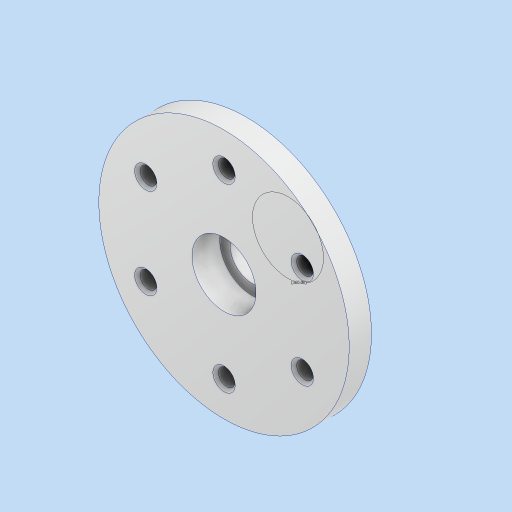
# Autodesk Inventor part: output pin holder
Saved by Autodesk Inventor 2023 (Build 270158000, 158)
## iProperties
Created: 2023-01-17
Part Number: output pin holder
Material: Aluminum 6061
Document SubType Name: Modeling
Designer: caden
Density: 2.7 g/cm^3
Appearance: Aluminum - Flat
Mass: 151.84 g
Surface Area: 187.145 cm^2
Volume: 56.2372 cm^3
Description: 3D Print
Author: caden
Autodesk Inventor part; units mm, degrees
ref_plane "YZ Plane" through (0, 0, 0) normal (1, 0, 0) x (0, 1, 0)
ref_plane "XZ Plane" through (0, 0, 0) normal (0, 1, 0) x (-1, 0, 0)
ref_plane "XY Plane" through (0, 0, 0) normal (0, 0, 1) x (1, 0, 0)
ref_plane "Work Plane1" through (0, 0, 2.9972) normal (0, 0, 1) x (1, 0, 0)
sketch "Sketch1" plane through (0, 0, 2.9972) normal (0, 0, 1) x (1, 0, 0)
  circle A0 centre (0, 0) radius 17.4625
  circle A1 centre (0, 0) radius 32.5 construction
  circle A2 centre (0, 0) radius 45
  circle A3 centre (0, -32.5) radius 3
  circle A4 centre (28.1458, -16.25) radius 3
  circle A5 centre (28.1458, 16.25) radius 3
  circle A6 centre (0, 32.5) radius 3
  circle A7 centre (-28.1458, 16.25) radius 3
  circle A8 centre (-28.1458, -16.25) radius 3
  dimension "d1" = 65
  dimension "d0" = 34.925
  dimension "d2" = 90
  dimension "d3" = 6
  dimension "d6" = 360
  constraints: 8 centre point, 3 coincident, 1 vertical alignment, 15 other
  measures "d0" diameter of A0
  measures "d2" diameter of A2
  measures "d3" diameter of A3
extrude "Extrusion1" add sketch "Sketch1" along normal blind 8 contours A0 | A2
ref_plane "Work Plane2" through (-75, -75, -12) normal (0, 0, -1) x (0, 1, 0)
extrude "Extrusion2" add sketch "Sketch1" against normal blind 15 contours A0
sketch "Sketch4" plane through (0, 0, 10.9972) normal (0, 0, 1) x (1, 0, 0)
  point P0 (0, 0)
  point P1 (0, 0)
  constraints: 1 coincident
hole "Hole1" at (0, 0, 10.9972) direction (0, 0, -1) diameter 15.5 end through all counterbore diameter 23 counterbore depth 10
chamfer "Chamfer1" distance 1 angle 45 6 edges at (-3, 32.5, 10.9972) (25.1458, 16.25, 10.9972) (25.1458, -16.25, 10.9972) (-3, -32.5, 10.9972) (-31.1458, -16.25, 10.9972) (-31.1458, 16.25, 10.9972)
sketch "Sketch5" plane through (0, 0, -12.0028) normal (0, 0, -1) x (-1, 0, 0)
  circle A0 centre (0, 0) radius 12.75 construction
  line L0 (-12.75, 0) -> (0, 0) construction
  dimension "d37" = 25.5
  constraints: 2 end point, 1 coincident, 1 horizontal, 1 horizontal alignment, 2 other
hole "Hole2" at (12.75, 0, -12.0028) direction (0, 0, 1) diameter 6.5 depth 6 countersink diameter 7 countersink angle 90
pattern_circular "Circular Pattern1" count 5 over 360 about axis through (0, 0, 2.9972) along (0, 0, -1) of "Hole2"
sketch "Sketch6" plane through (0, 0, -12.0028) normal (0, 0, -1) x (-1, 0, 0)
  circle A0 centre (-3.94, -12.126) radius 3.25 projected
  circle A1 centre (0, 0) radius 12.75
  circle A2 centre (-3.94, -12.126) radius 3.5 projected
  line L0 (-3.94, -12.126) -> (-12.2467, -9.4269)
  line L1 (10.315, -7.4943) -> (5.1811, -14.5604)
  line L2 (10.315, 7.4943) -> (15.4488, 0.4281)
  line L3 (-3.94, 12.126) -> (4.3668, 14.825)
  line L4 (-12.75, 0) -> (-12.75, 8.7342)
  line L5 (0, 0) -> (10.315, -7.4943) construction
  dimension "d43" = 360
  constraints: 12 end point, 1 coincident, 20 other
body "Solid1"
